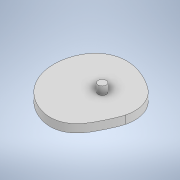
# Autodesk Inventor part: 凸輪_2
Saved by Autodesk Inventor 2022 (Build 260153000, 153)
## iProperties
Created: 2023-04-10
Part Number: 凸輪_2
Material: 一般
Document SubType Name: Modeling
Designer: JOU
Density: 1 g/cm^3
Appearance: 預設
Author: JOU
Autodesk Inventor part; units mm, degrees
ref_plane "YZ Plane" through (0, 0, 0) normal (1, 0, 0) x (0, 1, 0)
ref_plane "XZ Plane" through (0, 0, 0) normal (0, 1, 0) x (-1, 0, 0)
ref_plane "XY Plane" through (0, 0, 0) normal (0, 0, 1) x (1, 0, 0)
sketch "草圖1" plane through (0, 0, 0) normal (0, 1, 0) x (-1, 0, 0)
  spline S0 degree 5 number of poles 3605
  spline S1 degree 5 number of poles 3605
  point P0 (0, 0)
  point P1 (0, 0)
  point P2 (0, 0)
  constraints: 2 other
sketch "草圖1 outline for 擠出1" plane through (0, 0, 0) normal (0, 1, 0) x (-1, 0, 0)
  spline S0 degree 5 poles (-38.814091, 9.667801) (-37.954787, 13.117795) (-36.679851, 16.609751) (-35.157787, 20.092738) (-33.554322, 23.624015) (-30.192275, 30.685759) (-28.433626, 34.218594) (-26.610697, 37.713633) (-24.568657, 41.09884) (-19.892392, 47.415156) (-17.259175, 50.34605) (-14.244895, 52.93442) (-10.862578, 55.016233) (-3.549229, 58.034433) (0.383036, 58.971538) (4.502155, 59.262906) (8.667267, 58.949361) (13.850628, 57.924477) (14.886, 57.687752) (15.919249, 57.420864) (16.94955, 57.125398) (18.489347, 56.641713) (19.001534, 56.473802) (19.513048, 56.299256) (20.023668, 56.118339) (21.041408, 55.744726) (21.548154, 55.55213) (22.052688, 55.353781) (22.554924, 55.149712) (25.054171, 54.100938) (27.015277, 53.170723) (28.932814, 52.152117) (30.801502, 51.047923) (36.245182, 47.486992) (39.658434, 44.782751) (42.815289, 41.77484) (45.68121, 38.496164) (53.320542, 27.965442) (57.136233, 20.018331) (59.44821, 11.453956) (60.150121, 2.666272) (59.065011, -8.120807) (58.749578, -10.268304) (58.336873, -12.400012) (57.82803, -14.510064) (56.922263, -17.633853) (56.596839, -18.667951) (56.247309, -19.69521) (55.875141, -20.714695) (55.086103, -22.7266) (54.668814, -23.720265) (54.228118, -24.700467) (53.763378, -25.666032) (51.31627, -30.414798) (48.965283, -33.95991) (46.185837, -37.170516) (42.999043, -39.939087) (35.980938, -44.476986) (32.149104, -46.246771) (28.075656, -47.456641) (23.893019, -48.107011) (15.500513, -48.407309) (11.290186, -48.056887) (7.165373, -47.261781) (3.178261, -46.128161) (-4.508845, -43.3557) (-8.208006, -41.716466) (-11.754301, -39.911668) (-15.165982, -38.000018) (-20.000119, -34.938263) (-21.564424, -33.885646) (-23.075199, -32.797825) (-24.522673, -31.669532) (-26.236521, -30.199375) (-26.574524, -29.902366) (-26.907548, -29.602287) (-27.235382, -29.299042) (-27.880248, -28.686029) (-28.197545, -28.375949) (-28.510698, -28.061289) (-28.819853, -27.741906) (-29.73321, -26.771726) (-30.324141, -26.108019) (-30.896511, -25.428092) (-31.449731, -24.73264) (-34.11715, -21.181257) (-35.935738, -18.102942) (-37.403372, -14.835146) (-38.496236, -11.430894) (-39.55535, -6.207313) (-39.811718, -4.446509) (-39.969962, -2.673288) (-40.029433, -0.894914) (-39.970719, 1.769375) (-39.92647, 2.656927) (-39.857612, 3.543023) (-39.764217, 4.426755) (-39.528494, 6.187672) (-39.386278, 7.064497) (-39.219392, 7.938598) (-39.028917, 8.805302) (-38.814091, 9.667801) knots 0 0 0 0 0 0 0.0625 0.0625 0.0625 0.0625 0.125 0.125 0.125 0.125 0.1875 0.1875 0.1875 0.1875 0.25 0.25 0.25 0.25 0.265625 0.265625 0.265625 0.265625 0.2734375 0.2734375 0.2734375 0.2734375 0.28125 0.28125 0.28125 0.28125 0.3125 0.3125 0.3125 0.3125 0.375 0.375 0.375 0.375 0.5 0.5 0.5 0.5 0.53125 0.53125 0.53125 0.53125 0.546875 0.546875 0.546875 0.546875 0.5625 0.5625 0.5625 0.5625 0.625 0.625 0.625 0.625 0.6875 0.6875 0.6875 0.6875 0.75 0.75 0.75 0.75 0.8125 0.8125 0.8125 0.8125 0.84375 0.84375 0.84375 0.84375 0.8515625 0.8515625 0.8515625 0.8515625 0.859375 0.859375 0.859375 0.859375 0.875 0.875 0.875 0.875 0.9375 0.9375 0.9375 0.9375 0.96875 0.96875 0.96875 0.96875 0.984375 0.984375 0.984375 0.984375 1 1 1 1 1 1
extrude "擠出1" add sketch "草圖1 outline for 擠出1" along normal blind 10
sketch "草圖2" plane through (0, 10, 0) normal (0, 1, 0) x (1, 0, 0)
  circle A0 centre (0, 0) radius 5
  dimension "d2" = 10
  constraints: 1 centre point, 1 coincident
  measures "d2" diameter of A0
extrude "擠出2" add sketch "草圖2" along normal blind 10
